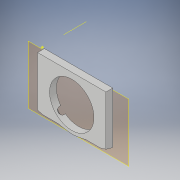
# Autodesk Inventor part: 20_Cube_Insert_Kinematic_Mirrormount_45_Thorlabsadapter
Saved by Autodesk Inventor 2019 (Build 230136000, 136)
## iProperties
Created: 2019-10-30
Part Number: 20_Cube_Insert_Kinematic_Mirrormount_45_Thorlabsadapter
Material: Generic
Document SubType Name: Modeling
Designer: diederichbenedict
Density: 1 g/cm^3
Appearance: Default
Author: diederichbenedict
Autodesk Inventor part; units mm, degrees
ref_plane "Work Plane1" through (0, -12.9, 0) normal (0, 0, 1) x (1, 0, 0)
sketch "Sketch1" plane through (0, -12.9, 0) normal (0, 0, 1) x (1, 0, 0)
  circle A0 centre (26.812722, 14) radius 1.4 construction
  line L0 (6.812722, 27.5) -> (46.812722, 27.5)
  line L1 (46.812722, 27.5) -> (46.812722, 0.5)
  line L2 (46.812722, 0.5) -> (6.812722, 0.5)
  line L3 (6.812722, 0.5) -> (6.812722, 27.5)
  line L4 (6.812722, 27.5) -> (46.812722, 0.5) construction
  line L5 (46.812722, 27.5) -> (6.812722, 0.5) construction
  circle A1 centre (26.812722, 14) radius 12.7 construction
  circle A2 centre (26.812722, 14) radius 13
  line L6 (6.812722, 27.5) -> (46.812722, 27.5)
  line L7 (46.812722, 27.5) -> (46.812722, 30.5)
  line L8 (46.812722, 30.5) -> (6.812722, 30.5)
  line L9 (6.812722, 30.5) -> (6.812722, 27.5)
  point P0 (0, 12.9)
  dimension "d0" = 40
  dimension "d1" = 27
  dimension "d2" = 0.3
  dimension "d14" = 3
  constraints: 20 end point, 4 parallel, 2 horizontal, 2 midpoint, 2 perpendicular, 1 centre point
  measures "d0" distance of L1.end L2.end
  measures "d1" distance of L0.end L1.end
  measures "d2" radial gap between concentric circles of A1 A2
  measures "d14" distance of L7.end L6.end
ref_plane "Work Plane2" through (14.362722, 1.55, 6) normal (0, 0, 1) x (1, 0, 0)
sketch "Sketch1 outline for Extrusion1" plane through (0, -12.9, 0) normal (0, 0, 1) x (1, 0, 0)
  line L0 (6.812722, 30.5) -> (6.812722, 0.5)
  line L1 (46.812722, 0.5) -> (6.812722, 0.5)
  line L2 (46.812722, 0.5) -> (46.812722, 30.5)
  line L3 (46.812722, 30.5) -> (6.812722, 30.5)
  circle A0 centre (26.812722, 14) radius 13
extrude "Extrusion1" add sketch "Sketch1 outline for Extrusion1" along normal up to surface (6 mm away)
ref_plane "Work Plane3" through (16.812722, -12.4, 0) normal (-1, 0, 0) x (0, 0, 1)
sketch "Sketch6" plane through (6.812722, 17.6, 6) normal (0, 0, 1) x (1, 0, 0)
  circle A0 centre (20, -16.5) radius 13 projected
  point P0 (-6.812722, -17.6)
extrude "Extrusion5" [suppressed]
sketch "Sketch2 outline for Revolution1" plane through (16.812722, -12.4, 0) normal (-1, 0, 0) x (0, 0, 1)
  arc A0 (0.7, 21.053641) -> (0.7, 25.946359) centre (0.833518, 23.5) cw
  line L0 (0.7, 25.946359) -> (0.7, 21.053641)
revolve "Revolution1" cut sketch "Sketch2 outline for Revolution1" angle 360 about axis through (16.812722, 8.653641, 0.7) along (0, 1, 0)
pattern_linear "Rectangular Pattern1" count 2 spacing 20 along (0, -1, 0) count 2 spacing 20 along (1, 0, 0) of "Revolution1"
sketch "Sketch3" plane through (6.812722, -12.4, 6) normal (0, 0, 1) x (1, 0, 0)
  ellipse E0 centre (20, 24.3) end of major axis (41.071782, 24.3) minor radius 14.9 (7.319306, 12.4) -> (20, 9.4) ccw construction
  ellipse E1 centre (20, 24.3) end of major axis (41.071782, 24.3) minor radius 14.9 (20, 9.4) -> (32.680694, 12.4) ccw construction
  line L0 (40, 0) -> (0, 0) construction
  line L1 (40, 30) -> (40, 0) construction
  line L2 (0, 30) -> (40, 30) construction
  line L3 (0, 0) -> (0, 30) construction
  circle A0 centre (20, 13.5) radius 13 construction
  line L4 (40, 0) -> (0, 0)
  line L5 (10.000321, 0) -> (29.999679, 0)
  spline S0 degree 5 poles (2.302067, 2.9833) (5.546725, 1.254685) (9.033916, -0.018604) (12.64709, -0.852086) (16.323542, -1.269798) (20, -1.26991) knots 0 0 0 0 0 0 1 1 1 1 1 1
  spline S1 degree 5 poles (20, -1.26991) (23.676458, -1.269798) (27.35291, -0.852086) (30.966084, -0.018604) (34.453275, 1.254685) (37.697933, 2.9833) knots 0 0 0 0 0 0 1 1 1 1 1 1
  point P0 (-6.812722, 12.4)
  constraints: 2 end point, 2 point on line, 10 other
sketch "Sketch3 outline for Extrusion2" plane through (6.812722, -12.4, 6) normal (0, 0, 1) x (1, 0, 0)
  spline S0 degree 5 poles (10.000312, -0.000035) (11.956143, -0.511007) (13.946107, -0.891275) (15.957058, -1.143535) (17.978528, -1.269848) (20, -1.26991) knots 0 0 0 0 0 0 1 1 1 1 1 1
  line L0 (29.999679, 0) -> (10.000321, 0)
  spline S1 degree 5 poles (20, -1.26991) (22.021472, -1.269848) (24.042942, -1.143535) (26.053893, -0.891275) (28.043857, -0.511007) (29.999688, -0.000035) knots 0 0 0 0 0 0 1 1 1 1 1 1
extrude "Extrusion2" add sketch "Sketch3 outline for Extrusion2" against normal up to surface (6 mm away)
ref_plane "Work Plane4" through (26.812722, 23.9, 43.615113) normal (-0.7071068, 0, 0.7071068) x (-0.7071068, 0, -0.7071068)
sketch "Sketch4" plane through (26.812722, 23.9, 43.615113) normal (-0.7071068, 0, 0.7071068) x (-0.7071068, 0, -0.7071068)
  arc A0 (33.866605, 23.9) -> (15.933395, 23.9) centre (24.9, 12) ccw
  line L0 (12.455766, 36.3) -> (19.527061, 36.3) construction
  line L1 (12.455766, 6.3) -> (12.455766, 36.3) construction
  line L2 (40.740037, 6.3) -> (12.455766, 6.3) construction
  line L3 (40.740037, 36.3) -> (40.740037, 6.3) construction
  arc A1 (33.554545, 36.3) -> (9.129834, 32.41306) centre (24.9, 12) ccw
  line L4 (12.455766, 36.3) -> (40.740037, 36.3)
  line L5 (33.554545, 36.3) -> (40.740037, 36.3)
  line L6 (40.740037, 36.3) -> (40.740037, 42.517938)
  line L7 (40.740037, 42.517938) -> (9.28132, 42.969378)
  line L8 (9.28132, 42.969378) -> (9.129834, 32.41306)
  line L9 (33.668742, 36.3) -> (40.740037, 36.3)
  point P0 (49.8, 23.9)
  constraints: 8 end point, 2 perpendicular, 2 point on circle, 1 centre point, 1 horizontal, 2 other
sketch "Sketch4 outline for Extrusion3" plane through (26.812722, 23.9, 43.615113) normal (-0.7071068, 0, 0.7071068) x (-0.7071068, 0, -0.7071068)
  line L0 (33.554545, 36.3) -> (40.740037, 36.3)
  arc A0 (9.129834, 32.41306) -> (33.554545, 36.3) centre (24.9, 12) cw
  line L1 (9.28132, 42.969378) -> (9.129834, 32.41306)
  line L2 (40.740037, 42.517938) -> (9.28132, 42.969378)
  line L3 (40.740037, 36.3) -> (40.740037, 42.517938)
extrude "Extrusion3" cut sketch "Sketch4 outline for Extrusion3" against normal through all
ref_plane "Work Plane5" through (62.02664, 23.9, 8.401195) normal (0.7071068, 0, 0.7071068) x (-0.7071068, 0, 0.7071068)
sketch "Sketch5" plane through (62.02664, 23.9, 8.401195) normal (0.7071068, 0, 0.7071068) x (-0.7071068, 0, 0.7071068)
  arc A0 (33.866605, 23.9) -> (15.933395, 23.9) centre (24.9, 12) ccw
  arc A1 (40.472341, 32.666781) -> (9.327659, 32.666781) centre (24.9, 12) ccw
  line L0 (16.131258, 36.3) -> (11.888617, 36.3)
  line L1 (16.131258, 36.3) -> (16.244934, 36.386543) construction
  line L2 (16.244934, 36.386543) -> (16.131258, 36.3)
  line L3 (40.472341, 32.666781) -> (40.472341, 41.90235)
  line L4 (40.472341, 41.90235) -> (12.073171, 41.90235)
  line L5 (12.073171, 41.90235) -> (11.888617, 36.3)
  point P0 (37.918916, 23.9)
  constraints: 10 end point, 3 point on circle, 1 centre point, 1 collinear, 1 perpendicular, 1 vertical
sketch "Sketch5 outline for Extrusion4" plane through (62.02664, 23.9, 8.401195) normal (0.7071068, 0, 0.7071068) x (-0.7071068, 0, 0.7071068)
  arc A0 (40.472341, 32.666781) -> (16.244934, 36.386543) centre (24.9, 12) ccw
  line L0 (16.244934, 36.386543) -> (16.131258, 36.3)
  line L1 (16.131258, 36.3) -> (11.888617, 36.3)
  line L2 (11.888617, 36.3) -> (12.073171, 41.90235)
  line L3 (12.073171, 41.90235) -> (40.472341, 41.90235)
  line L4 (40.472341, 41.90235) -> (40.472341, 32.666781)
extrude "Extrusion4" cut sketch "Sketch5 outline for Extrusion4" against normal through all
sketch "Sketch7" plane through (6.812722, 17.6, 0) normal (0, 1, 0) x (1, 0, 0)
  line L0 (0, -6) -> (40, -6) construction
  line L1 (40, 0) -> (40, -6) construction
  line L2 (40, 0) -> (0, 0) construction
  line L3 (0, 0) -> (0, -6) construction
  line L4 (0, -6) -> (40, -6)
  line L5 (40, -6) -> (40, -4)
  line L6 (40, -4) -> (0, -4)
  line L7 (0, -4) -> (0, -6)
  point P0 (-6.812722, 0)
  dimension "d27" = 2
  constraints: 8 end point, 2 parallel, 1 horizontal, 1 perpendicular, 1 point on line
  measures "d27" distance between parallel lines of L0 L6
sketch "Sketch7 outline for Extrusion6" plane through (6.812722, 17.6, 0) normal (0, 1, 0) x (1, 0, 0)
  line L0 (0, -4) -> (0, -6)
  line L1 (40, -4) -> (0, -4)
  line L2 (40, -6) -> (40, -4)
  line L3 (0, -6) -> (40, -6)
extrude "Extrusion6" cut sketch "Sketch7 outline for Extrusion6" against normal through all
sketch "Sketch2" plane through (16.812722, -12.4, 0) normal (-1, 0, 0) x (0, 0, 1)
  line L0 (-7.227366, 36.4) -> (9.998822, 36.4)
  line L1 (0, 0.5) -> (0, 26.5)
  line L2 (-4.766482, 2) -> (6.826793, 2)
  line L3 (-4.055337, 5.704206) -> (7.537938, 5.704206)
  line L4 (-4.766482, 22) -> (6.826793, 22)
  line L5 (-4.055337, 25.704206) -> (7.537938, 25.704206)
  arc A0 (0.7, 25.946359) -> (0.7, 21.053641) centre (0.833518, 23.5) ccw
  arc A1 (0.7, 5.95) -> (0.7, 1.05) centre (0.7, 3.5) ccw
  line L6 (0.7, 1.05) -> (0.7, 5.95)
  line L7 (0.7, 21.053641) -> (0.7, 25.946359)
  line L8 (6, 0) -> (6, 30) construction
  line L9 (0, 30) -> (6, 30) construction
  line L10 (0, 30) -> (0, 0) construction
  line L11 (0, 0) -> (6, 0) construction
  point P0 (0, 12.4)
  dimension "d22" = 4.9
  dimension "d23" = 1.5
  dimension "d24" = 1.5
  dimension "d31" = 0.7
  dimension "d32" = 20
  dimension "d33" = 3.5
  dimension "d34" = 2.45
  constraints: 12 end point, 4 point on circle, 2 centre point, 2 collinear
  measures "d22" diameter of A1
  measures "d23" distance from line of L2 A1.centre
  measures "d24" distance from line of A0.centre L4
  measures "d31" distance between parallel lines of L10 L7
  measures "d32" vertical distance of A0.centre A1.centre
  measures "d33" distance from line of L11 A1.centre
  measures "d34" radius of A0
body "Solid1"
